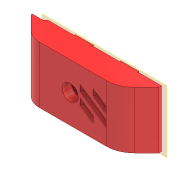
# Autodesk Inventor part: Cover
Saved by Autodesk Inventor 2021 (Build 250183000, 183)
## iProperties
Created: 2021-08-30
Part Number: Cover
Material: Generisch
Document SubType Name: Modeling
Designer: Rama
Density: 1 g/cm^3
Appearance: Hellrot
Author: Rama
Autodesk Inventor part; units mm, degrees
ref_plane "YZ Plane" through (0, 0, 0) normal (1, 0, 0) x (0, 1, 0)
ref_plane "XZ Plane" through (0, 0, 0) normal (0, 1, 0) x (-1, 0, 0)
ref_plane "XY Plane" through (0, 0, 0) normal (0, 0, 1) x (1, 0, 0)
sketch "Skizze1" plane through (0, 0, 0) normal (0, 0, 1) x (1, 0, 0)
  line L0 (-4.2865, -7.5) -> (-4.2865, -10) projected
  line L1 (5.2135, -10) -> (-4.2865, -10) projected
  line L2 (5.2135, -10) -> (5.2135, -7.5) projected
  arc A0 (11.7135, -7.5) -> (5.2135, -7.5) centre (8.4635, -7.5) ccw projected
  line L3 (11.7135, -7.5) -> (11.7135, -10) projected
  line L4 (20, -10) -> (11.7135, -10) projected
  line L5 (20, 10) -> (20, -10) projected
  line L6 (11.7135, 10) -> (20, 10) projected
  line L7 (11.7135, 10) -> (11.7135, 7.5) projected
  arc A1 (5.2135, 7.5) -> (11.7135, 7.5) centre (8.4635, 7.5) ccw projected
  line L8 (5.2135, 7.5) -> (5.2135, 10) projected
  line L9 (-4.2865, 10) -> (5.2135, 10) projected
  line L10 (-4.2865, 10) -> (-4.2865, 7.5) projected
  arc A2 (-10.7865, 7.5) -> (-4.2865, 7.5) centre (-7.5365, 7.5) ccw projected
  line L11 (-10.7865, 7.5) -> (-10.7865, 10) projected
  line L12 (-20, 10) -> (-10.7865, 10) projected
  line L13 (-20, -10) -> (-20, 10) projected
  line L14 (-10.7865, -10) -> (-20, -10) projected
  line L15 (-10.7865, -10) -> (-10.7865, -7.5) projected
  arc A3 (-4.2865, -7.5) -> (-10.7865, -7.5) centre (-7.5365, -7.5) ccw projected
  circle A4 centre (-7.5365, 7.5) radius 3.2
  circle A5 centre (8.4635, 7.5) radius 3.2
  circle A6 centre (8.4635, -7.5) radius 3.2
  circle A7 centre (-7.5365, -7.5) radius 3.2
  line L16 (-10.7365, 7.5) -> (-4.3365, 7.5)
  line L17 (-4.3365, 7.5) -> (-4.3365, 12.5)
  line L18 (-4.3365, 12.5) -> (-10.7365, 12.5)
  line L19 (-10.7365, 12.5) -> (-10.7365, 7.5)
  line L20 (5.2635, 7.5) -> (11.6635, 7.5)
  line L21 (11.6635, 7.5) -> (11.6635, 12.5)
  line L22 (11.6635, 12.5) -> (5.2635, 12.5)
  line L23 (5.2635, 12.5) -> (5.2635, 7.5)
  line L24 (-10.7365, -7.5) -> (-4.3365, -7.5)
  line L25 (-4.3365, -7.5) -> (-4.3365, -12.5)
  line L26 (-4.3365, -12.5) -> (-10.7365, -12.5)
  line L27 (-10.7365, -12.5) -> (-10.7365, -7.5)
  line L28 (5.2635, -7.5) -> (11.6635, -7.5)
  line L29 (11.6635, -7.5) -> (11.6635, -12.5)
  line L30 (11.6635, -12.5) -> (5.2635, -12.5)
  line L31 (5.2635, -12.5) -> (5.2635, -7.5)
  line L32 (20, 10) -> (-19.9, 10)
  line L33 (-19.9, 10) -> (-19.9, -10)
  line L34 (-19.9, -10) -> (20, -10)
  line L35 (20, -10) -> (20, 10)
  circle A8 centre (-3.95, 0) radius 2 projected
  point P0 (0, 0)
  point P1 (-4.3365, -7.5)
  point P2 (-10.7365, -10)
  point P3 (-4.3365, -10)
  point P4 (11.6635, -7.5)
  point P5 (5.2635, -10)
  point P6 (11.6635, -10)
  point P7 (11.6635, 7.5)
  point P8 (11.6635, 10)
  point P9 (5.2635, 10)
  point P10 (-10.7365, 10)
  point P11 (-4.3365, 7.5)
  point P12 (-4.3365, 10)
  dimension "d1" = 6.4
  dimension "d2" = 6.4
  dimension "d3" = 6.4
  dimension "d4" = 6.4
  dimension "d0" = 3.25
  dimension "d5" = 6.4
  dimension "d6" = 5
  dimension "d7" = 5
  dimension "d8" = 6.4
  dimension "d9" = 6.4
  dimension "d10" = 6.4
  dimension "d11" = 5
  dimension "d12" = 5
  dimension "d13" = 0.1
  constraints: 40 end point, 10 parallel, 5 horizontal, 5 perpendicular, 4 coincident, 1 point on line, 12 other
  measures "d0" radius of A2
  measures "d5" distance of L17.end L18.end
  measures "d6" distance of L18.end L16.start
  measures "d7" distance of L22.end L20.start
  measures "d8" distance of L21.end L22.end
  measures "d9" distance of L25.end L26.end
  measures "d10" distance of L29.end L30.end
  measures "d11" distance of L30.end L28.start
  measures "d12" distance of L26.end L24.start
  measures "d13" distance between parallel lines of L13 L33
extrude "Extrusion1" add sketch "Skizze1" against normal blind 0.4 contours L34 A7 L25 | L31 A6 L34 | L24 A7 | A7 L34 L24 | L27 A7 L34 | L28 A6 L34 | A6 L28 | L29 L34 A6 | L32 A4 L19 | L16 A4 | A4 L32 L16 | A4 L32 L17 | L21 A5 L32 | L20 A5 L32 | A5 L20 | L32 A5 L23
ref_plane "Arbeitsebene1" through (0, 0, 0) normal (0, 0, 1) x (1, 0, 0)
sketch "Skizze2" plane through (0, 0, 0) normal (0, 0, 1) x (1, 0, 0)
  line L0 (-4.2865, -7.5) -> (-4.2865, -10) projected
  line L1 (5.2135, -10) -> (-4.2865, -10) projected
  line L2 (5.2135, -10) -> (5.2135, -7.5) projected
  arc A0 (11.7135, -7.5) -> (5.2135, -7.5) centre (8.4635, -7.5) ccw projected
  line L3 (11.7135, -7.5) -> (11.7135, -10) projected
  line L4 (20, -10) -> (11.7135, -10) projected
  line L5 (20, 10) -> (20, -10) projected
  line L6 (11.7135, 10) -> (20, 10) projected
  line L7 (11.7135, 10) -> (11.7135, 7.5) projected
  arc A1 (5.2135, 7.5) -> (11.7135, 7.5) centre (8.4635, 7.5) ccw projected
  line L8 (5.2135, 7.5) -> (5.2135, 10) projected
  line L9 (-4.2865, 10) -> (5.2135, 10) projected
  line L10 (-4.2865, 10) -> (-4.2865, 7.5) projected
  arc A2 (-10.7865, 7.5) -> (-4.2865, 7.5) centre (-7.5365, 7.5) ccw projected
  line L11 (-10.7865, 7.5) -> (-10.7865, 10) projected
  line L12 (-20, 10) -> (-10.7865, 10) projected
  line L13 (-20, -10) -> (-20, 10) projected
  line L14 (-10.7865, -10) -> (-20, -10) projected
  line L15 (-10.7865, -10) -> (-10.7865, -7.5) projected
  arc A3 (-4.2865, -7.5) -> (-10.7865, -7.5) centre (-7.5365, -7.5) ccw projected
  line L16 (20, 10) -> (-19.9, 10)
  line L17 (-19.9, 10) -> (-19.9, -10)
  line L18 (-19.9, -10) -> (20, -10)
  line L19 (20, -10) -> (20, 10)
  circle A4 centre (-3.95, 0) radius 2 projected
  point P0 (0, 0)
  dimension "d16" = 0.1
  constraints: 8 end point, 2 parallel, 1 horizontal, 1 perpendicular, 1 point on line
  measures "d16" distance between parallel lines of L13 L17
extrude "Extrusion2" add sketch "Skizze2" along normal blind 7.9 contours A3 L15 L14 L17 L12 L11 A2 L10 L9 L8 A1 L7 L6 L5 L4 L3 A0 L2 L1 L0 | L0 L18 L15 A3 | L2 A0 L3 L18 | L16 L10 A2 L11 | L7 A1 L8 L16 | A4
chamfer "Fase1" distance 7 angle 45 1 edges at (20, 0, 7.9)
sketch "Skizze3" plane through (5.2635, 10, -0.4) normal (0, 1, 0) x (1, 0, 0)
  line L0 (-31.7635, -2.7) -> (-34.2635, -0.2) projected
  line L1 (-30.2635, -1.2) -> (-26.0635, -1.2) projected
  line L2 (-25.2635, -0.4) -> (-26.0635, -1.2) projected
  line L3 (-34.2635, -0.2) -> (-26.1635, -8.3)
  line L4 (-34.2635, -0.2) -> (-22.8084, -0.2) construction
  line L5 (-25.1635, -8.3) -> (7.7365, -8.3) projected
  line L6 (-22, -8.3) -> (-26.1635, -8.3)
  line L7 (-25.1635, -0.4) -> (-25.1635, -8.3) projected
  line L8 (-33.2135, -1.25) -> (-26.0428, -1.25)
  line L9 (-26.0428, -1.25) -> (-25.1928, -0.4)
  line L10 (-26.0428, -1.25) -> (-24.8407, -1.25) construction
  line L11 (-25.1635, -0.4) -> (-25.1928, -0.4)
  line L12 (-32.8135, -1.65) -> (-32.8135, -1.25)
  point P0 (-5.2635, -0.4)
  dimension "d22" = 45
  dimension "d23" = 0.05
  dimension "d24" = 45
  dimension "d25" = 0.05
  dimension "d26" = 0.4
  constraints: 16 end point, 10 point on line, 3 horizontal, 2 equal length, 1 collinear, 1 parallel, 1 vertical
  measures "d22" angle of L3 L4
  measures "d23" distance between parallel lines of L1 L8
  measures "d24" angle of L10 L9
  measures "d25" distance from line of L2.start L9
  measures "d26" distance of L12.start L12.end
extrude "Extrusion3" add sketch "Skizze3" against normal up to surface (20 mm away) contours L0 L12 L8 L9 L11 L7 L6 L3
move faces "Verschieben1" translate (0, 0, 0.2) faces at (-9.6, 3.3333, 7.9)
fillet "Rundung1" radius 10 2 edges at (-20.7, 0, 8.1) (12.8, 0, 8.1)
sketch "Skizze4" plane through (-16.5579, 10, 8.1) normal (0, 0, 1) x (1, 0, 0)
  line L0 (25.2157, 0) -> (25.2157, -20) projected
  line L1 (25.2157, 0) -> (0, 0) projected
  line L2 (0, -20) -> (0, 0) projected
  line L3 (0, -20) -> (25.2157, -20) projected
  line L4 (20.6695, -15.213) -> (16.1232, -12.1176)
  line L5 (20.6695, -15.213) -> (26.1695, -15.213) construction
  line L6 (16.1232, -12.1176) -> (16.1232, -9.9176)
  line L7 (16.1232, -9.9176) -> (20.6695, -13.013)
  line L8 (20.6695, -13.013) -> (20.6695, -15.213)
  line L9 (25.2157, -14.1954) -> (16.1232, -8.0046)
  line L10 (16.1232, -8.0046) -> (16.1232, -5.8046)
  line L11 (16.1232, -5.8046) -> (25.2157, -11.9954)
  line L12 (25.2157, -14.1954) -> (25.2157, -11.9954)
  line L13 (25.2157, -10.0824) -> (20.6695, -6.987)
  line L14 (20.6695, -6.987) -> (20.6695, -4.787)
  line L15 (20.6695, -4.787) -> (25.2157, -7.8824)
  line L16 (25.2157, -7.8824) -> (25.2157, -10.0824)
  line L17 (16.1232, -15.213) -> (25.2157, -15.213)
  line L18 (25.2157, -15.213) -> (25.2157, -4.787)
  line L19 (25.2157, -4.787) -> (16.1232, -4.787)
  line L20 (16.1232, -4.787) -> (16.1232, -15.213)
  line L21 (0, -20) -> (0, 0) projected
  line L22 (0, -20) -> (12.6079, -20)
  line L23 (12.6079, -20) -> (12.6079, -10)
  line L24 (12.6079, -10) -> (0, -10)
  line L25 (0, -10) -> (0, -20)
  circle A0 centre (12.6079, -10) radius 2.8
  point P0 (16.5579, -10)
  dimension "d97" = 145.75
  dimension "d99" = 2.2
  dimension "d102" = 1.913
  dimension "d103" = 5.5
  dimension "d104" = 11
  dimension "d106" = 0
  dimension "d110" = 2.2
  dimension "d111" = 11
  dimension "d113" = 2.2
  dimension "d114" = 5.5
  dimension "d118" = 0
  dimension "d119" = 1.913
  dimension "d124" = 9.0925
  dimension "d125" = 10.4261
  dimension "d126" = 25.2157
  dimension "d127" = 20
  dimension "d128" = 0
  dimension "d129" = 4.787
  dimension "d146" = 20
  dimension "d147" = 10
  dimension "d148" = 12.6079
  dimension "d149" = 5.6
  constraints: 42 end point, 11 parallel, 3 horizontal, 3 vertical, 2 midpoint, 2 perpendicular, 2 point on line, 1 centre point, 1 coincident, 1 equal length
  measures "d97" angle of L5 L4
  measures "d99" distance of L4.end L6.end
  measures "d102" distance of L9.end L6.end
  measures "d103" distance of L4.start L4.end
  measures "d104" distance of L9.start L9.end
  measures "d106" distance from line of L9.end L6
  measures "d110" distance of L9.end L10.end
  measures "d111" distance of L10.end L11.end
  measures "d113" distance of L14.start L14.end
  measures "d114" distance of L13.start L14.start
  measures "d118" distance from line of L13.start L12
  measures "d119" distance of L13.start L11.end
  measures "d124" distance of L17.start L17.end
  measures "d125" distance of L19.end L17.start
  measures "d126" distance of L2.start L0.end
  measures "d127" distance of L0.start L0.end
  measures "d128" distance between parallel lines of L0 L18
  measures "d129" distance between parallel lines of L1 L19
  measures "d146" distance of L2.start L1.end
  measures "d147" distance of L22.end L23.end
  measures "d148" distance of L23.end L24.end
  measures "d149" diameter of A0
extrude "Extrusion4" cut sketch "Skizze4" against normal blind 1 contours L0 L13 L14 L15 | L0 L9 L10 L11 | L7 L8 L4 L6
sketch "Skizze5" plane through (-16.5579, 10, 8.1) normal (0, 0, 1) x (1, 0, 0)
  line L0 (25.2157, 0) -> (25.2157, -7.8824) projected
  line L1 (25.2157, 0) -> (0, 0) projected
  line L2 (0, -20) -> (0, 0) projected
  line L3 (0, -20) -> (25.2157, -20) projected
  line L4 (0, -20) -> (25.2157, -20) projected
  line L5 (0, -20) -> (12.6079, -20)
  line L6 (12.6079, -20) -> (12.6079, -10)
  line L7 (12.6079, -10) -> (0, -10)
  line L8 (0, -10) -> (0, -20)
  line L9 (25.2157, -14.1954) -> (25.2157, -20) projected
  line L10 (25.2157, -10.0824) -> (25.2157, -11.9954) projected
  line L11 (16.1232, -5.8046) -> (25.2157, -11.9954) projected
  line L12 (25.2157, -10.0824) -> (20.6695, -6.987) projected
  line L13 (20.6695, -6.987) -> (20.6695, -4.787) projected
  line L14 (20.6695, -4.787) -> (25.2157, -7.8824) projected
  line L15 (25.2157, -14.1954) -> (16.1232, -8.0046) projected
  line L16 (16.1232, -8.0046) -> (16.1232, -5.8046) projected
  point P0 (16.5579, -10)
  dimension "d135" = 25.2157
  dimension "d136" = 20
  dimension "d137" = 12.6079
  dimension "d138" = 10
  constraints: 8 end point, 2 parallel, 1 horizontal, 1 perpendicular
  measures "d135" distance of L2.start L3.end
  measures "d136" distance of L2.start L1.end
  measures "d137" distance of L7.end L6.end
  measures "d138" distance of L6.end L5.end
hole "Bohrung1" at (-3.95, 0, 8.1) direction (0, 0, -1) diameter 3.2 end through all counterbore diameter 5.6 counterbore depth 3.2 clearance for "Inbusschraube ISO 4762" size "M3" standard "ISO"
chamfer "Fase3" distance 0.8 angle 45 12 edges at (8.6579, 1.0176, 7.1) (6.3847, 1.4653, 7.1) (4.1116, 4.113, 7.1) (6.3847, 3.6653, 7.1) (8.6579, -3.0954, 7.1) (4.1116, -1.1, 7.1) (4.1116, 1.1, 7.1) (-0.4346, 3.0954, 7.1) (1.8385, -1.4653, 7.1) (4.1116, -4.113, 7.1) (1.8385, -3.6653, 7.1) (-0.4346, -1.0176, 7.1)
delete faces "Fläche löschen1" heal yes whole lump no faces at (-19.7723, 3.3333, 7.5693) (-26.243, -3.3333, 2.557)
sketch "Skizze8" plane through (-4.3365, 10, 0) normal (0, 1, 0) x (1, 0, 0)
  line L0 (-20.6635, -0.8) -> (-22.2535, 0.7899) projected
  line L1 (-23.5398, 2.0762) -> (-12.3017, -9.1618)
  line L2 (12.9943, -8.1) -> (-23.2135, -8.1) projected
  line L3 (-23.2135, -0.85) -> (-23.2135, -8.1) projected
  line L4 (-16.4428, -0.85) -> (-23.2135, -0.85) projected
  line L5 (-20.2135, -1.25) -> (-20.2135, -0.85)
  point P0 (4.3365, 0)
  point P1 (-7.9648, -8.1)
  point P2 (-13.3635, -8.1)
  dimension "d167" = 0
  dimension "d168" = 0.4
  constraints: 4 end point, 2 point on line, 1 collinear, 1 vertical
  measures "d167" distance between parallel lines of L0 L1
  measures "d168" distance of L5.start L5.end
extrude "Extrusion7" cut sketch "Skizze8" against normal through all
fillet "Rundung4" radius 7 1 edges at (-17.7, 0, 8.1)
equation "\"d2\" = d1"
equation "\"d3\" = d1"
equation "\"d4\" = d1"
equation "\"d5\" = d1"
equation "\"d7\" = d6"
equation "\"d8\" = d1"
equation "\"d9\" = d1"
equation "\"d10\" = d9"
equation "\"d11\" = d6"
equation "\"d12\" = d6"
